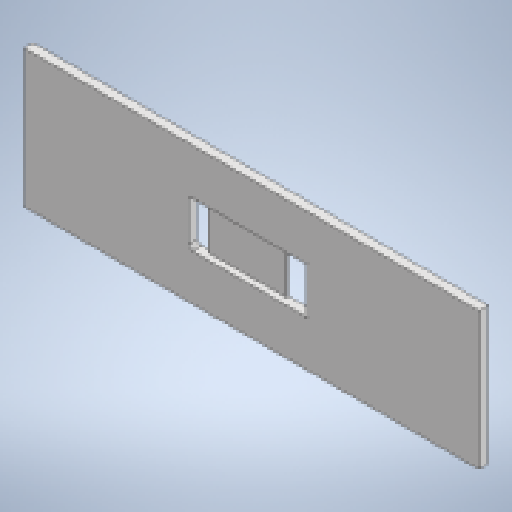
# Autodesk Inventor part: backplate-0
Saved by Autodesk Inventor 2023 (Build 270158030, 158C)
## iProperties
Created: 2024-09-24
Part Number: backplate-0
Material: Generic
Document SubType Name: Modeling
Designer: Imogen Heard
Density: 1 g/cm^3
Appearance: Default
Author: Imogen Heard
Autodesk Inventor part; units mm, degrees
ref_plane "YZ Plane" through (0, 0, 0) normal (1, 0, 0) x (0, 1, 0)
ref_plane "XZ Plane" through (0, 0, 0) normal (0, 1, 0) x (-1, 0, 0)
ref_plane "XY Plane" through (0, 0, 0) normal (0, 0, 1) x (1, 0, 0)
sketch "Sketch1" plane through (0, 0, 0) normal (0, 0, 1) x (1, 0, 0)
  line L0 (34.0626, 1) -> (0, 1) projected
  line L1 (34.0626, 14) -> (34.0626, 1) projected
  line L2 (0, 14) -> (34.0626, 14) projected
  line L3 (0, 1) -> (0, 14) projected
  arc A0 (1.6411, 15) -> (0, 14) centre (6, 6) ccw projected
  line L4 (0, 14) -> (34.0626, 14) projected
  line L5 (34.0626, 15) -> (34.0626, 14) projected
  line L6 (34.0626, 15) -> (1.6411, 15) projected
  line L7 (1.6411, 0) -> (34.0626, 0) projected
  arc A1 (0, 1) -> (1.6411, 0) centre (6, 9) ccw projected
  line L8 (1.6411, 0) -> (34.0626, 0) projected
  line L9 (34.0626, 0) -> (34.0626, 1) projected
  line L10 (34.0626, 1) -> (0, 1) projected
  line L11 (-53.669, 30) -> (95.331, 30)
  line L12 (95.331, 30) -> (95.331, -15)
  line L13 (95.331, -15) -> (-53.669, -15)
  line L14 (-53.669, -15) -> (-53.669, 30)
  line L15 (70.331, 1) -> (64.4317, 1) projected
  arc A2 (70.331, 1) -> (70.331, 14) centre (70.331, 7.5) ccw projected
  line L16 (64.4317, 14) -> (70.331, 14) projected
  line L17 (64.4317, 1) -> (64.4317, 14) projected
  arc A3 (70.331, 0) -> (70.331, 15) centre (70.331, 7.5) ccw projected
  line L18 (-22.7698, 1) -> (-28.669, 1) projected
  line L19 (-22.7698, 14) -> (-22.7698, 1) projected
  line L20 (-28.669, 14) -> (-22.7698, 14) projected
  arc A4 (-28.669, 14) -> (-28.669, 1) centre (-28.669, 7.5) ccw projected
  arc A5 (-28.669, 15) -> (-28.669, 0) centre (-28.669, 7.5) ccw projected
  line L21 (34.0626, 1) -> (41.6619, 1) projected
  line L22 (41.6619, 14) -> (34.0626, 14) projected
  line L23 (34.0626, 15) -> (41.004, 15) projected
  line L24 (41.004, 0) -> (34.0626, 0) projected
  line L25 (41.6619, 1) -> (41.6619, 14) projected
  line L26 (34.0626, 15) -> (39.0626, 15)
  line L27 (39.0626, 15) -> (39.0626, 0)
  line L28 (39.0626, 0) -> (34.0626, 0)
  line L29 (34.0626, 0) -> (34.0626, 15)
  point P0 (0, 0)
  point P1 (20.831, 30)
  dimension "d0" = 15
  dimension "d1" = 15
  dimension "d2" = 25
  dimension "d3" = 25
  dimension "d11" = 5
  constraints: 16 end point, 4 parallel, 2 horizontal, 2 perpendicular, 1 midpoint
  measures "d0" distance from line of point (20.831, 30) L6
  measures "d1" distance between parallel lines of L13 L7
  measures "d2" distance from line of L14 A4.centre
  measures "d3" distance from line of A2.centre L12
  measures "d11" distance between parallel lines of L27 L9
extrude "Extrusion1" add sketch "Sketch1" against normal blind 3 contours L27 L22 L25 L21 | L11 L12 L13 L14 | L15 L17 L16 A2 | L18 A4 L20 L19
sketch "Sketch2" plane through (1.6411, 0, 0) normal (0, 1, 0) x (1, 0, 0)
  arc A0 (32.4215, 0) -> (40.0208, 3.5) centre (32.4215, 10) ccw projected
  line L0 (32.4215, 0) -> (-1.6411, 0) projected
  arc A1 (4.3589, 2) -> (0, 1) centre (4.3589, -8) ccw projected
  line L1 (1.1287, 3.5) -> (30.0208, 3.5) projected
  line L2 (30.0208, 2) -> (4.3589, 2) projected
  line L3 (0, 3) -> (37.4215, 3) projected
  line L4 (2.8589, 3) -> (28.5208, 3)
  line L5 (28.5208, 3) -> (28.5208, 2.2)
  line L6 (28.5208, 2.2) -> (2.8589, 2.2)
  line L7 (2.8589, 2.2) -> (2.8589, 3)
  line L8 (30.0208, 4.5) -> (30.0208, 2) projected
  point P0 (32.4215, 3)
  dimension "d6" = 1.5
  dimension "d7" = 0.2
  dimension "d8" = 1.5
  constraints: 8 end point, 2 parallel, 1 horizontal, 1 perpendicular, 1 point on line
  measures "d6" distance between parallel lines of L5 L8
  measures "d7" distance between parallel lines of L2 L6
  measures "d8" distance from line of L2.end L7
extrude "Extrusion2" add sketch "Sketch2" along normal up to surface (15 mm away)
chamfer "Chamfer1" distance 3 angle 45 1 edges at (39.0626, 7.5, -3)
fillet "Fillet1" radius 12 4 edges at (95.331, 30, -1.5) (95.331, -15, -1.5) (-53.669, -15, -1.5) (-53.669, 30, -1.5)
sketch "Sketch3" plane through (0, 0, -3) normal (0, 0, -1) x (-1, 0, 0)
  circle A0 centre (45.669, -7) radius 1.55
  circle A1 centre (45.669, 22) radius 1.55
  circle A2 centre (-87.331, -7) radius 1.55
  circle A3 centre (-87.331, 22) radius 1.55
  line L0 (-83.331, -15) -> (41.669, -15) projected
  line L1 (53.669, -3) -> (53.669, 18) projected
  line L2 (41.669, 30) -> (-83.331, 30) projected
  line L3 (-95.331, 18) -> (-95.331, -3) projected
  point P0 (0, 0)
  dimension "d16" = 3.1
  dimension "d17" = 8
  dimension "d18" = 8
  dimension "d19" = 8
  dimension "d20" = 8
  constraints: 4 centre point, 3 equal radius, 2 horizontal alignment, 2 vertical alignment
  measures "d16" diameter of A0
  measures "d17" distance from line of L0 A0.centre
  measures "d18" distance from line of L1 A0.centre
  measures "d19" distance from line of A1.centre L2
  measures "d20" distance from line of A2.centre L3
extrude "Extrusion3" cut sketch "Sketch3" against normal through all
chamfer "Chamfer2" distance 2 angle 45 8 edges at (20.831, -15, -3) (-50.1543, -11.4853, -3) (-53.669, 7.5, -3) (-50.1543, 26.4853, -3) (20.831, 30, -3) (91.8162, 26.4853, -3) (95.331, 7.5, -3) (91.8162, -11.4853, -3)
equation "\"d18\" = d17"
equation "\"d19\" = d17"
equation "\"d20\" = d17"
